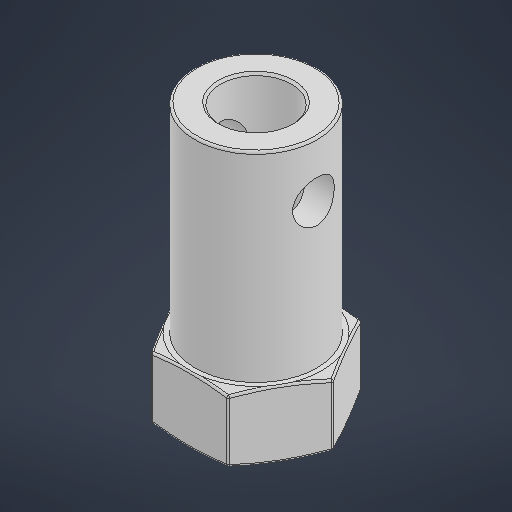
# Autodesk Inventor part: 짧은 나사
Saved by Autodesk Inventor 2026.1 (Build 301233020, 233B)
## iProperties
Created: 2025-10-29
Part Number: 짧은 나사
Material: 일반
Document SubType Name: Modeling
Designer: jaewook
Density: 1 g/cm^3
Appearance: 기본값
Author: jaewook
Autodesk Inventor part; units mm, degrees
ref_plane "YZ Plane" through (0, 0, 0) normal (1, 0, 0) x (0, 1, 0)
ref_plane "XZ Plane" through (0, 0, 0) normal (0, 1, 0) x (-1, 0, 0)
ref_plane "XY Plane" through (0, 0, 0) normal (0, 0, 1) x (1, 0, 0)
sketch "스케치1" plane through (0, 0, 0) normal (0, 1, 0) x (-1, 0, 0)
  line L0 (-3.4641, 6) -> (3.4641, 6)
  line L1 (3.4641, 6) -> (6.9282, 0)
  line L2 (6.9282, 0) -> (3.4641, -6)
  line L3 (3.4641, -6) -> (-3.4641, -6)
  line L4 (-3.4641, -6) -> (-6.9282, 0)
  line L5 (-6.9282, 0) -> (-3.4641, 6)
  point P0 (0, 0)
  point P1 (0, 0)
  dimension "d4" = 12
  constraints: 12 end point, 1 coincident, 1 horizontal, 13 other
  measures "d4" distance between parallel lines of L0 L3
extrude "돌출1" add sketch "스케치1" along normal blind 6
sketch "스케치2" plane through (0, 6, 0) normal (0, 1, 0) x (1, 0, 0)
  circle A0 centre (0, 0) radius 5.5
  dimension "d3" = 11
  constraints: 1 centre point, 1 coincident
  measures "d3" diameter of A0
extrude "돌출2" add sketch "스케치2" along normal blind 18
sketch "스케치3" plane through (0, 24, 0) normal (0, 1, 0) x (1, 0, 0)
  circle A0 centre (0, 0) radius 5.5 projected
hole "구멍1" at (0, 24, 0) direction (0, -1, 0) diameter 3.75 end through all counterbore diameter 6.4 counterbore depth 18
sketch "스케치4" plane through (0, 0, 0) normal (1, 0, 0) x (0, 1, 0)
  circle A0 centre (19, 0) radius 1.875
  line L0 (24, -5.5) -> (24, 5.5) projected
  point P0 (0, 0)
  dimension "d14" = 3.75
  dimension "d15" = 5
  constraints: 1 centre point, 1 horizontal alignment
  measures "d14" diameter of A0
  measures "d15" distance from line of A0.centre L0
extrude "돌출3" cut sketch "스케치4" along normal mid plane 24
sketch "스케치5" plane through (0, 0, 0) normal (0, 0, 1) x (1, 0, 0)
  line L0 (-3.4641, 0) -> (-6.9282, 0) projected
  line L1 (-6.9282, 0) -> (-6.9282, 6) projected
  line L2 (-3.4641, 6) -> (-6.9282, 6) projected
  line L3 (-3.4641, 0) -> (-3.4641, 6) projected
  line L4 (-5.9282, 6) -> (-6.9282, 5.7321)
  line L5 (-6.9282, 0) -> (-6.9282, 6) projected
  line L6 (-6.9282, 0.2679) -> (-5.9282, 0)
  line L7 (-3.4641, 6) -> (-6.9282, 6) projected
  line L8 (-5.9282, 6) -> (-6.9282, 6)
  line L9 (-6.9282, 6) -> (-6.9282, 5.7321)
  line L10 (-5.9282, 6) -> (-6.9282, 6)
  line L11 (0, -6) -> (0, 36) projected
  point P0 (0, 0)
  dimension "d18" = 15
  dimension "d20" = 1
  dimension "d21" = 1
  dimension "d22" = 15
  constraints: 10 end point, 4 point on line, 2 collinear, 1 perpendicular
  measures "d18" angle of L4 L2
  measures "d20" distance of L1.end L4.start
  measures "d21" distance of L0.end L6.end
  measures "d22" angle of L0 L6
revolve "회전1" cut sketch "스케치5" angle 360 about axis through (0, -10, 0) along (0, 1, 0) contours L0 L1 L6 | L4 L1 L2
chamfer "모따기1" distance 0.2 angle 45 1 edges at (0, 0, -1.875)
fillet "모깎기1" radius 0.2 18 edges at (3.4641, 3, 6) (6.9282, 3, 0) (3.4641, 3, -6) (-3.4641, 3, -6) (-6.9282, 3, 0) (-3.4641, 3, 6) (-5.1962, 0.0192, 3) (-5.1962, 5.9808, 3) (0, 5.9808, 6) (0, 0.0192, 6) (5.1962, 0.0192, 3) (5.1962, 5.9808, 3) (5.1962, 5.9808, -3) (5.1962, 0.0192, -3) (0, 0.0192, -6) (0, 5.9808, -6) (-5.1962, 0.0192, -3) (-5.1962, 5.9808, -3)
chamfer "모따기2" distance 0.2 angle 45 1 edges at (0, 24, -3.2)
fillet "모깎기2" radius 0.2 1 edges at (-5.5, 24, 0)
